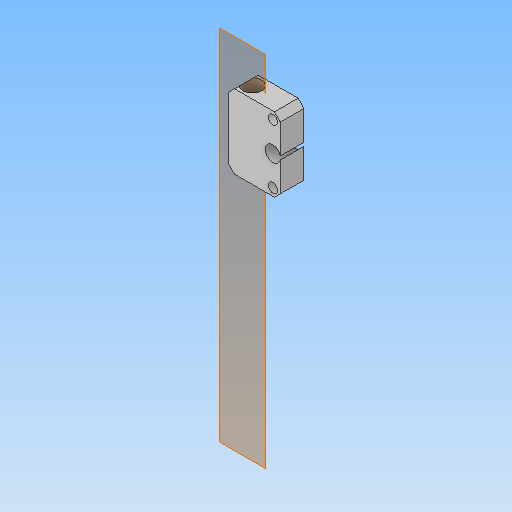
# Autodesk Inventor part: 06_OPENTRONS_Microscope_Extraslide_slide
Saved by Autodesk Inventor 2019.4 (Build 234330000, 330)
## iProperties
Created: 2020-11-19
Part Number: 06_OPENTRONS_Microscope_Extraslide_slide
Material: Generic
Document SubType Name: Modeling
Designer: diederichbenedict
Density: 1 g/cm^3
Appearance: Default
Author: diederichbenedict
Autodesk Inventor part; units mm, degrees
ref_plane "YZ Plane" through (0, 0, 0) normal (1, 0, 0) x (0, 1, 0)
ref_plane "XZ Plane" through (0, 0, 0) normal (0, 1, 0) x (-1, 0, 0)
ref_plane "XY Plane" through (0, 0, 0) normal (0, 0, 1) x (1, 0, 0)
ref_plane "Work Plane1" through (0, 0, 0) normal (0, 0, 1) x (1, 0, 0)
sketch "Sketch1" plane through (0, 0, 0) normal (0, 0, 1) x (1, 0, 0)
  circle A0 centre (-10.1084, -16.6095) radius 3 construction
  circle A1 centre (-10.1084, -56.6095) radius 3 construction
  circle A2 centre (-10.1084, -36.6095) radius 5.15 projected
  line L0 (-29.1084, -220.5) -> (-29.1084, 29.5)
  line L1 (-35.1084, -220.5) -> (-35.1084, 29.5)
  line L2 (-40.1084, -61.6095) -> (-5.1084, -61.6095)
  line L3 (-5.1084, -61.6095) -> (-5.1084, -11.6095)
  line L4 (-5.1084, -11.6095) -> (-40.1084, -11.6095)
  line L5 (-40.1084, -11.6095) -> (-40.1084, -61.6095)
  line L6 (-40.1084, -61.6095) -> (-5.1084, -11.6095) construction
  line L7 (-5.1084, -61.6095) -> (-40.1084, -11.6095) construction
  circle A3 centre (-10.1084, -16.6095) radius 3.1
  circle A4 centre (-10.1084, -56.6095) radius 3.1
  point P0 (0, 0)
  point P1 (-22.6084, -36.6095)
  point P2 (-5.1084, -35.3756)
  point P3 (-5.1084, -37.8434)
  dimension "d0" = 35
  dimension "d1" = 50
  dimension "d2" = 5
  dimension "d3" = 6.2
  dimension "d4" = 6.2
  constraints: 16 end point, 2 centre point, 2 coincident, 2 midpoint, 2 parallel, 2 point on circle, 2 point on line, 2 vertical, 1 horizontal, 1 perpendicular, 4 other
  measures "d0" distance of L4.end L3.end
  measures "d1" distance of L3.end L2.end
  measures "d2" distance from line of A2.centre L3
  measures "d3" diameter of A3
  measures "d4" diameter of A4
extrude "Extrusion1" add sketch "Sketch1" along normal mid plane 16 contours A2 L3 L2 L0 L4 | L0 L2 L1 L4 | L1 L2 L5 L4
sketch "Sketch2" plane through (-40.1084, -61.6095, 8) normal (0, -1, 0) x (1, 0, 0)
  circle A0 centre (8, -8) radius 6 projected
  circle A1 centre (8, -8) radius 6.3
  point P0 (40.1084, -8)
  dimension "d7" = 0.3
  constraints: 1 centre point
  measures "d7" radial gap between concentric circles of A0 A1
extrude "Extrusion2" cut sketch "Sketch2" against normal through all contours A0 | A1
chamfer "Chamfer1" distance 4 angle 45 4 edges at (-5.1084, -61.6095, 0) (-5.1084, -11.6095, 0) (-40.1084, -61.6095, 0) (-40.1084, -11.6095, 0)
body "Solid1"
